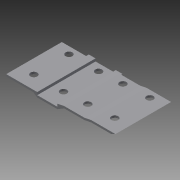
# Autodesk Inventor part: Finger_Support_base_Screwing
Saved by Autodesk Inventor 2015 (Build 190159000, 159)
## iProperties
Created: 2016-09-14
Part Number: Finger_Support_base_Screwing
Material: Generic
Document SubType Name: Modeling
Designer: Neelotpal Nag
Density: 1 g/cm^3
Appearance: Default
Author: Neelotpal Nag
Autodesk Inventor part; units mm, degrees
ref_plane "YZ Plane" through (0, 0, 0) normal (1, 0, 0) x (0, 1, 0)
ref_plane "XZ Plane" through (0, 0, 0) normal (0, 1, 0) x (-1, 0, 0)
ref_plane "XY Plane" through (0, 0, 0) normal (0, 0, 1) x (1, 0, 0)
sketch "Sketch1" plane through (0, 0, 0) normal (0, 0, 1) x (1, 0, 0)
  line L0 (0, 0) -> (81, 0)
  line L1 (0, 0) -> (0, -41.25)
  line L2 (0, -41.25) -> (81, -41.25)
  line L3 (81, -41.25) -> (81, 0)
  line L4 (23, 0) -> (23, 2)
  line L5 (23, 2) -> (38, 2)
  line L6 (38, 2) -> (38, 0)
  line L7 (3, 0) -> (3, -41.25)
  line L8 (18, 0) -> (18, -41.25)
  line L9 (23, 0) -> (23, -41.25)
  line L10 (38, 0) -> (38, -41.25)
  line L11 (43, 0) -> (43, -41.25)
  line L12 (58, 0) -> (58, -41.25)
  line L13 (63, 0) -> (63, -41.25)
  line L14 (78, 0) -> (78, -41.25)
  line L15 (0, 0) -> (3, 0)
  line L16 (3, 0) -> (3, -41.25)
  line L17 (3, -41.25) -> (0, -41.25)
  line L18 (0, -41.25) -> (0, 0)
  line L19 (78, 0) -> (81, 0)
  line L20 (81, 0) -> (81, -41.25)
  line L21 (81, -41.25) -> (78, -41.25)
  line L22 (78, -41.25) -> (78, 0)
  circle A0 centre (10.5, -5.25) radius 2.5
  circle A1 centre (10.5, -31.248) radius 2.5
  circle A2 centre (30.5, -3.25) radius 2.5
  circle A3 centre (30.5, -29.248) radius 2.5
  circle A4 centre (50.5, -5.25) radius 2.5
  circle A5 centre (50.5, -31.248) radius 2.5
  circle A6 centre (70.5, -5.25) radius 2.5
  circle A7 centre (70.5, -31.248) radius 2.5
  point P0 (10.5, -41.25)
  point P1 (50.5, 0)
  point P2 (70.5, 0)
  point P3 (30.5, 0)
  dimension "d0" = 81
  dimension "d2" = 41.25
  dimension "d3" = 2
  dimension "d24" = 5
  dimension "d25" = 5
  dimension "d26" = 5
  dimension "d27" = 5
  dimension "d28" = 5
  dimension "d29" = 5
  dimension "d30" = 5
  dimension "d31" = 5
  constraints: 42 end point, 11 vertical, 10 coincident, 8 centre point, 5 parallel, 3 horizontal, 3 perpendicular, 26 other
  measures "d0" distance of point (0, 0) point (81, 0)
  measures "d2" distance of L1.start L1.end
  measures "d3" distance of L4.start L4.end
  measures "d24" diameter of A0
  measures "d25" diameter of A1
  measures "d26" diameter of A2
  measures "d27" diameter of A3
  measures "d28" diameter of A4
  measures "d29" diameter of A5
  measures "d30" diameter of A6
  measures "d31" diameter of A7
sketch "Sketch3" plane through (0, 0, 0) normal (0, 1, 0) x (-1, 0, 0)
  line L0 (0, 0) -> (-81, 0) projected
  line L1 (-23, 0) -> (-38, 0) projected
  line L2 (0, 0) -> (-81, 0) projected
  line L3 (-23, 0) -> (-23, -2)
  line L4 (-23, -2) -> (-38, -2)
  line L5 (-38, -2) -> (-38, 0)
  line L6 (-43, 0) -> (-43, 1)
  line L7 (-43, 1) -> (-58, 1)
  line L8 (-58, 1) -> (-58, 0)
  line L9 (-63, 0) -> (-63, 2)
  line L10 (-63, 2) -> (-78, 2)
  line L11 (-78, 2) -> (-78, 0)
  line L12 (-23, -2) -> (-38, -2)
  line L13 (-38, -2) -> (-38, -3.5)
  line L14 (-38, -3.5) -> (-23, -3.5)
  line L15 (-23, -3.5) -> (-23, -2)
  line L16 (-18, 0) -> (-23, -3.5)
  line L17 (-38, -3.5) -> (-43, 0)
  line L18 (-43, 1) -> (-58, 1)
  line L19 (-58, 1) -> (-58, -0.5)
  line L20 (-58, -0.5) -> (-43, -0.5)
  line L21 (-43, -0.5) -> (-43, 1)
  line L22 (-38, 0) -> (-43, 1)
  line L23 (-63, 2) -> (-78, 2)
  line L24 (-78, 2) -> (-78, 0.5)
  line L25 (-78, 0.5) -> (-63, 0.5)
  line L26 (-63, 0.5) -> (-63, 2)
  line L27 (-58, 1) -> (-63, 2)
  line L28 (-58, -0.5) -> (-63, 0.5)
  line L29 (-78, 2) -> (-81, 2)
  line L30 (-81, 2) -> (-78, 0.5)
  line L31 (-43, 1) -> (-38, 0)
  line L32 (-43, 0) -> (-43, 1)
  line L33 (-43, 0) -> (-38, 0)
  line L34 (-38, 0) -> (-43, 1)
  line L35 (-43, 1) -> (-43, 0)
  line L36 (-38, -3.5) -> (-43, -0.5)
  line L37 (-43, -0.5) -> (-58, -0.5)
  line L38 (-58, 1) -> (-58, -0.5)
  line L39 (-58, 1) -> (-43, 1)
  line L40 (-58, -0.5) -> (-58, 1)
  line L41 (-58, 1) -> (-63, 2)
  line L42 (-63, 2) -> (-63, 0.5)
  line L43 (-63, 0.5) -> (-58, -0.5)
  line L44 (-58, -0.5) -> (-60.5, 0)
  line L45 (-58, -0.5) -> (-58, 0)
  line L46 (-58, 0) -> (-60.5, 0)
  line L47 (-60.5, 0) -> (-63, 0.5)
  line L48 (-63, 0.5) -> (-63, 2)
  line L49 (-63, 2) -> (-58, 1)
  line L50 (-58, 1) -> (-58, -0.5)
  point P0 (-3, 0)
  dimension "d4" = 2
  dimension "d5" = 1
  dimension "d6" = 2
  dimension "d7" = 15
  dimension "d8" = 90
  dimension "d11" = 1.5
  dimension "d16" = 15
  dimension "d17" = 1.5
  constraints: 96 end point, 9 parallel, 9 perpendicular, 7 collinear, 6 horizontal, 4 vertical, 1 midpoint, 1 point on line, 2 other
  measures "d4" distance of L3.start L3.end
  measures "d5" distance of L6.start L6.end
  measures "d6" distance of L9.start L9.end
  measures "d7" distance of L9.end L10.end
  measures "d8" angle of L10 L9
  measures "d11" distance of L13.end L12.end
  measures "d16" distance of L20.end L19.end
  measures "d17" distance of L19.end L18.end
extrude "Extrusion1" add sketch "Sketch1" against normal blind 1.5 contours L0 L7 L2 L1 | L0 L8 L2 L7 | L0 L9 L2 L8 | A0 | A1
extrude "Extrusion2" add sketch "Sketch3" against normal blind 41.25 contours L16 L15 L3 L0 | L14 L13 L4 L15 | L5 L13 L17 L0
extrude "Extrusion3" add sketch "Sketch3" along normal blind 2 contours L16 L15 L3 L0 | L14 L13 L4 L15 | L5 L13 L17 L0
extrude "Extrusion4" add sketch "Sketch3" against normal blind 41.25 contours L0 L6 L22 | L36 L21 L17 | L21 L20 L19 L0 | L0 L8 L7 L6 | L9 L25 L11 L10 | L11 L30 L29
extrude "Extrusion5" add sketch "Sketch3" against normal blind 41.25 contours L19 L28 L0 | L0 L28 L9 L27 L8
extrude "Extrusion6" cut sketch "Sketch1" along normal through all both and the other way through all contours A0 | A1 | A2 | A3 | A4 | A5 | A6 | A7
body "Solid1"
